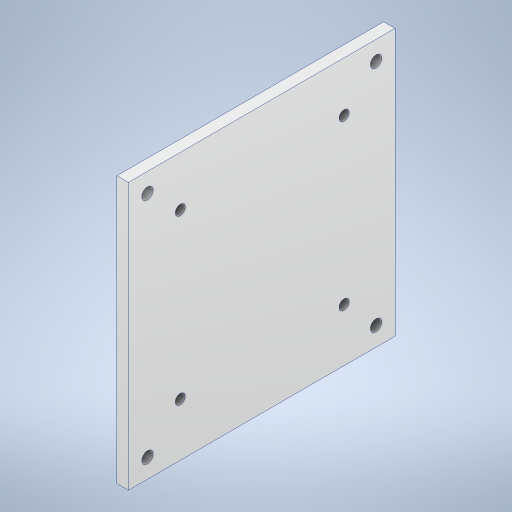
# Autodesk Inventor part: lidar_plate
Saved by Autodesk Inventor 2023 (Build 270158000, 158)
## iProperties
Created: 2023-01-12
Part Number: lidar_plate
Material: Aluminum 6061
Document SubType Name: Sheet Metal
Designer: LAB-505
Density: 2.74922 g/cm^3
Sheet Metal Rule: Default
Appearance: Aluminum - Flat
Mass: 40 g
Surface Area: 107.523 cm^2
Volume: 14.5496 cm^3
Author: LAB-505
Autodesk Inventor part; units mm, degrees
ref_plane "YZ Plane" through (0, 0, 0) normal (1, 0, 0) x (0, 1, 0)
ref_plane "XZ Plane" through (0, 0, 0) normal (0, 1, 0) x (-1, 0, 0)
ref_plane "XY Plane" through (0, 0, 0) normal (0, 0, 1) x (1, 0, 0)
sketch "Sketch1" plane through (0, 0, 0) normal (1, 0, 0) x (0, 1, 0)
  line L0 (8.5457, 136.9798) -> (8.5457, 103.4797)
  spline S0 degree 3 poles (19.375, 147.8091) (18.6641, 147.8091) (17.9599, 147.7397) (17.2623, 147.601) (16.5652, 147.4624) (15.8881, 147.2569) (15.2308, 146.9847) (14.5742, 146.7128) (13.9501, 146.3792) (13.3586, 145.984) (12.7676, 145.5892) (12.2206, 145.1402) (11.7175, 144.6372) (11.215, 144.1347) (10.766, 143.5877) (10.3708, 142.9962) (9.9759, 142.4053) (9.6423, 141.7812) (9.37, 141.1239) (9.098, 140.4674) (8.8926, 139.7902) (8.7538, 139.0925) (8.6151, 138.3952) (8.5457, 137.691) (8.5457, 136.9798) knots 0 0 0 0 0.125 0.125 0.125 0.25 0.25 0.25 0.375 0.375 0.375 0.5 0.5 0.5 0.625 0.625 0.625 0.75 0.75 0.75 0.875 0.875 0.875 1 1 1 1
  line L1 (52.875, 147.8091) -> (19.375, 147.8091)
  arc A0 (58.801, 146.0438) -> (54.8456, 147.6282) centre (52.875, 136.9798) ccw
  ellipse E0 centre (52.881, 136.9737) end of major axis (52.8771, 126.1401) minor radius 10.825 (61.939, 142.9057) -> (58.801, 146.0438) ccw
  line L2 (63.7043, 103.4798) -> (63.7043, 136.9798)
  spline S1 degree 3 poles (58.801, 94.4157) (59.4265, 94.8247) (60.0037, 95.2936) (60.5324, 95.8223) (61.061, 96.3507) (61.5298, 96.9279) (61.939, 97.5537) knots 0 0 0 0 0.5 0.5 0.5 1 1 1 1
  spline S2 degree 3 poles (52.875, 92.6505) (53.5374, 92.6505) (54.1943, 92.7107) (54.8456, 92.8313) knots 0 0 0 0 1 1 1 1
  line L3 (19.375, 92.6505) -> (52.875, 92.6505)
  spline S3 degree 3 poles (10.311, 97.5538) (10.72, 96.9282) (11.1888, 96.3511) (11.7175, 95.8223) (12.246, 95.2938) (12.8231, 94.825) (13.449, 94.4158) knots 0 0 0 0 0.5 0.5 0.5 1 1 1 1
  arc A1 (57.625, 140.4108) -> (57.625, 143.0488) centre (57.625, 141.7298) ccw
  arc A2 (57.625, 143.0488) -> (57.625, 140.4108) centre (57.625, 141.7298) ccw
  arc A3 (57.625, 97.4108) -> (57.625, 100.0488) centre (57.625, 98.7298) ccw
  arc A4 (57.625, 100.0488) -> (57.625, 97.4108) centre (57.625, 98.7298) ccw
  arc A5 (14.625, 97.4108) -> (14.625, 100.0488) centre (14.625, 98.7298) ccw
  arc A6 (14.625, 100.0488) -> (14.625, 97.4108) centre (14.625, 98.7298) ccw
  circle A7 centre (14.625, 141.7298) radius 1.319
  arc A8 (63.5235, 138.9504) -> (61.939, 142.9057) centre (52.875, 136.9798) ccw
  line L4 (0, 0) -> (70, 0)
  line L5 (70, 0) -> (70, -70)
  line L6 (70, -70) -> (0, -70)
  line L7 (0, -70) -> (0, 0)
  point P0 (36.125, 120.2298)
  point P1 (63.5235, 101.5091)
  point P2 (62.9439, 99.4934)
  point P3 (56.8613, 93.4109)
  point P4 (57.625, 142.7363)
  dimension "d0" = 70
  dimension "d1" = 70
  constraints: 16 end point, 16 point on circle, 9 centre point, 2 parallel, 1 horizontal, 1 perpendicular, 15 other
  measures "d0" distance of L5.end L6.end
  measures "d1" distance of L4.end L5.end
extrude "Extrusion1" add sketch "Sketch1" along normal blind 3 contours L4 L5 L6 L7
sketch "Sketch2" plane through (3, 0, 0) normal (1, 0, 0) x (0, 0, -1)
  line L0 (7.5282, 52.1652) -> (7.5282, 18.6652)
  spline S0 degree 3 poles (18.3575, 62.9945) (17.6466, 62.9945) (16.9424, 62.9251) (16.2448, 62.7864) (15.5477, 62.6478) (14.8706, 62.4424) (14.2133, 62.1702) (13.5567, 61.8982) (12.9326, 61.5646) (12.341, 61.1694) (11.7501, 60.7746) (11.2031, 60.3257) (10.7, 59.8227) (10.1975, 59.3201) (9.7485, 58.7731) (9.3533, 58.1816) (8.9584, 57.5907) (8.6248, 56.9666) (8.3525, 56.3094) (8.0805, 55.6528) (7.8751, 54.9756) (7.7363, 54.2779) (7.5976, 53.5807) (7.5282, 52.8764) (7.5282, 52.1652) knots 0 0 0 0 0.125 0.125 0.125 0.25 0.25 0.25 0.375 0.375 0.375 0.5 0.5 0.5 0.625 0.625 0.625 0.75 0.75 0.75 0.875 0.875 0.875 1 1 1 1
  line L1 (51.8575, 62.9945) -> (18.3575, 62.9945)
  arc A0 (57.7835, 61.2292) -> (53.8281, 62.8137) centre (51.8575, 52.1652) ccw
  ellipse E0 centre (51.8635, 52.1592) end of major axis (51.8596, 41.3255) minor radius 10.825 (60.9215, 58.0912) -> (57.7835, 61.2292) ccw
  line L2 (62.6868, 18.6652) -> (62.6868, 52.1652)
  spline S1 degree 3 poles (57.7835, 9.6012) (58.409, 10.0102) (58.9862, 10.479) (59.5149, 11.0077) (60.0434, 11.5362) (60.5123, 12.1133) (60.9215, 12.7392) knots 0 0 0 0 0.5 0.5 0.5 1 1 1 1
  spline S2 degree 3 poles (51.8575, 7.8359) (52.5199, 7.8359) (53.1768, 7.8962) (53.8281, 8.0167) knots 0 0 0 0 1 1 1 1
  line L3 (18.3575, 7.8359) -> (51.8575, 7.8359)
  spline S3 degree 3 poles (9.2935, 12.7392) (9.7025, 12.1137) (10.1713, 11.5365) (10.7, 11.0077) (11.2285, 10.4792) (11.8056, 10.0104) (12.4315, 9.6012) knots 0 0 0 0 0.5 0.5 0.5 1 1 1 1
  arc A1 (56.6075, 55.5962) -> (56.6075, 58.2342) centre (56.6075, 56.9152) ccw
  arc A2 (56.6075, 58.2342) -> (56.6075, 55.5962) centre (56.6075, 56.9152) ccw
  arc A3 (56.6075, 12.5962) -> (56.6075, 15.2342) centre (56.6075, 13.9152) ccw
  arc A4 (56.6075, 15.2342) -> (56.6075, 12.5962) centre (56.6075, 13.9152) ccw
  arc A5 (13.6075, 12.5962) -> (13.6075, 15.2342) centre (13.6075, 13.9152) ccw
  arc A6 (13.6075, 15.2342) -> (13.6075, 12.5962) centre (13.6075, 13.9152) ccw
  circle A7 centre (13.6075, 56.9152) radius 1.319
  arc A8 (62.506, 54.1358) -> (60.9215, 58.0912) centre (51.8575, 52.1652) ccw
  point P0 (0, 0)
  point P1 (35.1075, 35.4152)
  point P2 (62.506, 16.6946)
  point P3 (61.9264, 14.6789)
  point P4 (55.8438, 8.5963)
  point P5 (56.6075, 57.9217)
  constraints: 16 point on circle, 9 centre point, 8 end point, 15 other
extrude "Extrusion2" cut sketch "Sketch2" against normal blind 68.4375
sketch "Sketch3" plane through (3, 0, 0) normal (1, 0, 0) x (0, 0, -1)
  circle A0 centre (5, 5) radius 1.5
  circle A1 centre (5, 65) radius 1.5
  circle A2 centre (65, 65) radius 1.5
  circle A3 centre (65, 5) radius 1.5
  point P0 (0, 0)
  dimension "d6" = 3
  dimension "d7" = 3
  dimension "d8" = 3
  dimension "d9" = 3
  constraints: 4 centre point
  measures "d6" diameter of A0
  measures "d7" diameter of A1
  measures "d8" diameter of A2
  measures "d9" diameter of A3
extrude "Extrusion3" cut sketch "Sketch3" against normal blind 39.5125
equation "\"BendRadius\" = Thickness"
equation "\"BendReliefWidth\" = Thickness"
equation "\"BendReliefDepth\" = 0.5 * Thickness"
equation "\"CornerReliefSize\" = 4 * Thickness"
equation "\"MinimumRemnant\" = 2 * Thickness"
equation "\"TransitionRadius\" = BendRadius"
equation "\"JacobiRadiusSize\" = BendRadius"
equation "\"GapSize\" = Thickness"
equation "\"Thickness\" = 3.048"
body "Solid1"
